Autodesk Fusion 360 part; units mm, degrees
note: some values were not read from the file. Set by a fixed rule: which sketch regions a step uses.
(part 4 of 10)
  spline S19 degree 5 poles (-4.5069, -15.3521) (-4.5055, -15.3505) (-4.5027, -15.3473) (-4.4985, -15.3425) (-4.493, -15.3361) (-4.486, -15.3281) (-4.4791, -15.3201) (-4.4722, -15.3121) (-4.4654, -15.3042) (-4.4586, -15.2962) (-4.4518, -15.2883) (-4.445, -15.2803) (-4.4383, -15.2724) (-4.4316, -15.2645) (-4.4249, -15.2565) (-4.4183, -15.2486) (-4.4117, -15.2407) (-4.4051, -15.2329) (-4.3985, -15.225) (-4.392, -15.2171) (-4.3855, -15.2093) (-4.3791, -15.2014) (-4.3726, -15.1936) (-4.3662, -15.1858) (-4.3599, -15.178) (-4.3535, -15.1702) (-4.3472, -15.1624) (-4.3409, -15.1546) (-4.3347, -15.1468) (-4.3285, -15.1391) (-4.3223, -15.1313) (-4.3161, -15.1236) (-4.31, -15.1159) (-4.3039, -15.1082) (-4.2978, -15.1005) (-4.2918, -15.0928) (-4.2858, -15.0851) (-4.2798, -15.0775) (-4.2738, -15.0698) (-4.2679, -15.0622) (-4.262, -15.0546) (-4.2562, -15.047) (-4.2503, -15.0394) (-4.2445, -15.0318) (-4.2388, -15.0242) (-4.233, -15.0167) (-4.2273, -15.0092) (-4.2216, -15.0016) (-4.216, -14.9941) (-4.2104, -14.9866) (-4.2048, -14.9791) (-4.1992, -14.9717) (-4.1937, -14.9642) (-4.1882, -14.9568) (-4.1827, -14.9494) (-4.1773, -14.942) (-4.1719, -14.9346) (-4.1665, -14.9272) (-4.1612, -14.9198) (-4.1559, -14.9125) (-4.1506, -14.9052) (-4.1453, -14.8978) (-4.1401, -14.8905) (-4.1349, -14.8833) (-4.1297, -14.876) (-4.1246, -14.8687) (-4.1195, -14.8615) (-4.1144, -14.8543) (-4.1094, -14.8471) (-4.1044, -14.8399) (-4.0994, -14.8328) (-4.0944, -14.8256) (-4.0895, -14.8185) (-4.0846, -14.8114) (-4.0798, -14.8043) (-4.0749, -14.7972) (-4.0701, -14.7901) (-4.0654, -14.7831) (-4.0606, -14.7761) (-4.0559, -14.7691) (-4.0512, -14.7621) (-4.0466, -14.7551) (-4.042, -14.7482) (-4.0374, -14.7413) (-4.0328, -14.7344) (-4.0283, -14.7275) (-4.0238, -14.7206) (-4.0193, -14.7138) (-4.0149, -14.707) (-4.0105, -14.7002) (-4.0061, -14.6934) (-4.0018, -14.6866) (-3.9974, -14.6799) (-3.9932, -14.6731) (-3.9889, -14.6665) (-3.9847, -14.6598) (-3.9805, -14.6531) (-3.9763, -14.6465) (-3.9722, -14.6399) (-3.9681, -14.6333) (-3.964, -14.6267) (-3.96, -14.6202) (-3.9559, -14.6137) (-3.952, -14.6072) (-3.948, -14.6007) (-3.9441, -14.5942) (-3.9402, -14.5878) (-3.9363, -14.5814) (-3.9325, -14.575) (-3.9287, -14.5687) (-3.9249, -14.5623) (-3.9212, -14.556) (-3.9175, -14.5497) (-3.9138, -14.5435) (-3.9101, -14.5373) (-3.9065, -14.5311) (-3.9029, -14.5249) (-3.8993, -14.5187) (-3.8958, -14.5126) (-3.8923, -14.5065) (-3.8888, -14.5004) (-3.8854, -14.4944) (-3.882, -14.4883) (-3.8786, -14.4824) (-3.8752, -14.4764) (-3.8719, -14.4704) (-3.8686, -14.4645) (-3.8654, -14.4587) (-3.8621, -14.4528) (-3.8589, -14.447) (-3.8558, -14.4412) (-3.8526, -14.4354) (-3.8495, -14.4297) (-3.8464, -14.424) (-3.8434, -14.4183) (-3.8403, -14.4126) (-3.8373, -14.407) (-3.8344, -14.4014) (-3.8314, -14.3959) (-3.8285, -14.3903) (-3.8257, -14.3848) (-3.8228, -14.3794) (-3.82, -14.3739) (-3.8172, -14.3685) (-3.8144, -14.3632) (-3.8117, -14.3578) (-3.809, -14.3525) (-3.8063, -14.3473) (-3.8037, -14.342) (-3.8011, -14.3368) (-3.7985, -14.3316) (-3.796, -14.3265) (-3.7934, -14.3214) (-3.791, -14.3163) (-3.7885, -14.3113) (-3.7861, -14.3063) (-3.7836, -14.3013) (-3.7813, -14.2964) (-3.7789, -14.2915) (-3.7766, -14.2867) (-3.7743, -14.2819) (-3.7721, -14.2771) (-3.7698, -14.2723) (-3.7676, -14.2676) (-3.7655, -14.263) (-3.7633, -14.2583) (-3.7612, -14.2537) (-3.7591, -14.2492) (-3.7571, -14.2447) (-3.755, -14.2402) (-3.753, -14.2358) (-3.7511, -14.2314) (-3.7491, -14.227) (-3.7472, -14.2227) (-3.7453, -14.2185) (-3.7435, -14.2142) (-3.7416, -14.21) (-3.7398, -14.2059) (-3.7381, -14.2018) (-3.7363, -14.1977) (-3.7346, -14.1937) (-3.7329, -14.1898) (-3.7313, -14.1858) (-3.7296, -14.1819) (-3.728, -14.1781) (-3.7265, -14.1743) (-3.7249, -14.1706) (-3.7234, -14.1669) (-3.7219, -14.1632) (-3.7204, -14.1596) (-3.719, -14.1561) (-3.7176, -14.1525) (-3.7162, -14.1491) (-3.7149, -14.1457) (-3.7136, -14.1423) (-3.7123, -14.139) (-3.711, -14.1357) (-3.7097, -14.1325) (-3.7085, -14.1293) (-3.7073, -14.1262) (-3.7062, -14.1232) (-3.7051, -14.1202) (-3.704, -14.1172) (-3.7029, -14.1143) (-3.7018, -14.1114) (-3.7008, -14.1086) (-3.6998, -14.1059) (-3.6988, -14.1032) (-3.6979, -14.1006) (-3.697, -14.098) (-3.6961, -14.0955) (-3.6952, -14.093) (-3.6944, -14.0906) (-3.6936, -14.0883) (-3.6928, -14.086) (-3.692, -14.0838) (-3.6913, -14.0816) (-3.6906, -14.0795) (-3.6899, -14.0775) (-3.6892, -14.0755) (-3.6886, -14.0736) (-3.688, -14.0717) (-3.6874, -14.0699) (-3.6869, -14.0682) (-3.6863, -14.0665) (-3.6858, -14.0649) (-3.6853, -14.0634) (-3.6849, -14.0619) (-3.6845, -14.0606) (-3.6841, -14.0592) (-3.6837, -14.058) (-3.6833, -14.0568) (-3.683, -14.0557) (-3.6827, -14.0546) (-3.6824, -14.0537) (-3.6821, -14.0528) (-3.6819, -14.0519) (-3.6817, -14.0512) (-3.6815, -14.0505) (-3.6813, -14.0499) (-3.6812, -14.0494) (-3.6811, -14.0491) (-3.681, -14.0488) (-3.681, -14.0487) (-3.681, -14.0486) knots -1 -1 -1 -1 -1 -1 -0.99583333 -0.99166667 -0.9875 -0.98333333 -0.97916667 -0.975 -0.97083333 -0.96666667 -0.9625 -0.95833333 -0.95416667 -0.95 -0.94583333 -0.94166667 -0.9375 -0.93333333 -0.92916667 -0.925 -0.92083333 -0.91666667 -0.9125 -0.90833333 -0.90416667 -0.9 -0.89583333 -0.89166667 -0.8875 -0.88333333 -0.87916667 -0.875 -0.87083333 -0.86666667 -0.8625 -0.85833333 -0.85416667 -0.85 -0.84583333 -0.84166667 -0.8375 -0.83333333 -0.82916667 -0.825 -0.82083333 -0.81666667 -0.8125 -0.80833333 -0.80416667 -0.8 -0.79583333 -0.79166667 -0.7875 -0.78333333 -0.77916667 -0.775 -0.77083333 -0.76666667 -0.7625 -0.75833333 -0.75416667 -0.75 -0.74583333 -0.74166667 -0.7375 -0.73333333 -0.72916667 -0.725 -0.72083333 -0.71666667 -0.7125 -0.70833333 -0.70416667 -0.7 -0.69583333 -0.69166667 -0.6875 -0.68333333 -0.67916667 -0.675 -0.67083333 -0.66666667 -0.6625 -0.65833333 -0.65416667 -0.65 -0.64583333 -0.64166667 -0.6375 -0.63333333 -0.62916667 -0.625 -0.62083333 -0.61666667 -0.6125 -0.60833333 -0.60416667 -0.6 -0.59583333 -0.59166667 -0.5875 -0.58333333 -0.57916667 -0.575 -0.57083333 -0.56666667 -0.5625 -0.55833333 -0.55416667 -0.55 -0.54583333 -0.54166667 -0.5375 -0.53333333 -0.52916667 -0.525 -0.52083333 -0.51666667 -0.5125 -0.50833333 -0.50416667 -0.5 -0.49583333 -0.49166667 -0.4875 -0.48333333 -0.47916667 -0.475 -0.47083333 -0.46666667 -0.4625 -0.45833333 -0.45416667 -0.45 -0.44583333 -0.44166667 -0.4375 -0.43333333 -0.42916667 -0.425 -0.42083333 -0.41666667 -0.4125 -0.40833333 -0.40416667 -0.4 -0.39583333 -0.39166667 -0.3875 -0.38333333 -0.37916667 -0.375 -0.37083333 -0.36666667 -0.3625 -0.35833333 -0.35416667 -0.35 -0.34583333 -0.34166667 -0.3375 -0.33333333 -0.32916667 -0.325 -0.32083333 -0.31666667 -0.3125 -0.30833333 -0.30416667 -0.3 -0.29583333 -0.29166667 -0.2875 -0.28333333 -0.27916667 -0.275 -0.27083333 -0.26666667 -0.2625 -0.25833333 -0.25416667 -0.25 -0.24583333 -0.24166667 -0.2375 -0.23333333 -0.22916667 -0.225 -0.22083333 -0.21666667 -0.2125 -0.20833333 -0.20416667 -0.2 -0.19583333 -0.19166667 -0.1875 -0.18333333 -0.17916667 -0.175 -0.17083333 -0.16666667 -0.1625 -0.15833333 -0.15416667 -0.15 -0.14583333 -0.14166667 -0.1375 -0.13333333 -0.12916667 -0.125 -0.12083333 -0.11666667 -0.1125 -0.10833333 -0.10416667 -0.1 -0.09583333 -0.09166667 -0.0875 -0.08333333 -0.07916667 -0.075 -0.07083333 -0.06666667 -0.0625 -0.05833333 -0.05416667 -0.05 -0.04583333 -0.04166667 -0.0375 -0.03333333 -0.02916667 -0.025 -0.02083333 -0.01666667 -0.0125 -0.00833333 -0.00416667 0 0 0 0 0 0
  arc A26 (8.5938, 10.7336) -> (7.5526, 11.49) centre (0, 0) ccw
  arc A27 (8.3931, 13.6219) -> (7.6003, 14.0796) centre (0, 0) ccw
  line L59 (2.3513, -14.3306) -> (2.2262, -13.5686)
  line L60 (9.0768, 11.3369) -> (9.0764, 11.3364)
  line L61 (11.235, 9.2016) -> (10.6376, 8.7123)
  line L62 (3.6808, -14.048) -> (3.681, -14.0486)
  arc A28 (10.6376, 8.7123) -> (9.7765, 9.6687) centre (0, 0) ccw
  line L63 (7.5526, 11.49) -> (7.9768, 12.1353)
  arc A29 (13.208, 9.0304) -> (12.6699, 9.771) centre (0, 0) ccw
  line L64 (0.6435, -13.7349) -> (0.6796, -14.5063)
  line L65 (10.3255, 10.2117) -> (10.326, 10.2121)
  spline S20 degree 5 poles (10.3616, 12.1917) (10.3596, 12.1908) (10.3558, 12.189) (10.35, 12.1863) (10.3423, 12.1828) (10.3327, 12.1783) (10.3231, 12.1738) (10.3136, 12.1693) (10.3041, 12.1648) (10.2946, 12.1603) (10.2852, 12.1558) (10.2758, 12.1513) (10.2664, 12.1468) (10.2571, 12.1423) (10.2478, 12.1378) (10.2385, 12.1332) (10.2292, 12.1287) (10.22, 12.1242) (10.2108, 12.1197) (10.2017, 12.1151) (10.1925, 12.1106) (10.1834, 12.1061) (10.1744, 12.1015) (10.1654, 12.097) (10.1564, 12.0924) (10.1474, 12.0879) (10.1385, 12.0834) (10.1296, 12.0788) (10.1207, 12.0743) (10.1119, 12.0697) (10.1031, 12.0651) (10.0943, 12.0606) (10.0855, 12.056) (10.0768, 12.0515) (10.0682, 12.0469) (10.0595, 12.0423) (10.0509, 12.0378) (10.0423, 12.0332) (10.0338, 12.0287) (10.0253, 12.0241) (10.0168, 12.0195) (10.0084, 12.015) (9.9999, 12.0104) (9.9916, 12.0058) (9.9832, 12.0013) (9.9749, 11.9967) (9.9666, 11.9921) (9.9584, 11.9876) (9.9502, 11.983) (9.942, 11.9785) (9.9338, 11.9739) (9.9257, 11.9693) (9.9176, 11.9648) (9.9096, 11.9602) (9.9016, 11.9557) (9.8936, 11.9511) (9.8857, 11.9465) (9.8777, 11.942) (9.8699, 11.9374) (9.862, 11.9329) (9.8542, 11.9283) (9.8464, 11.9238) (9.8387, 11.9193) (9.831, 11.9147) (9.8233, 11.9102) (9.8157, 11.9056) (9.8081, 11.9011) (9.8005, 11.8966) (9.793, 11.8921) (9.7855, 11.8875) (9.778, 11.883) (9.7706, 11.8785) (9.7632, 11.874) (9.7558, 11.8695) (9.7485, 11.865) (9.7412, 11.8605) (9.7339, 11.856) (9.7267, 11.8515) (9.7195, 11.847) (9.7124, 11.8425) (9.7053, 11.8381) (9.6982, 11.8336) (9.6912, 11.8291) (9.6841, 11.8247) (9.6772, 11.8202) (9.6702, 11.8158) (9.6633, 11.8113) (9.6565, 11.8069) (9.6496, 11.8025) (9.6428, 11.798) (9.6361, 11.7936) (9.6294, 11.7892) (9.6227, 11.7848) (9.616, 11.7804) (9.6094, 11.776) (9.6028, 11.7717) (9.5963, 11.7673) (9.5898, 11.7629) (9.5833, 11.7586) (9.5769, 11.7542) (9.5705, 11.7499) (9.5642, 11.7455) (9.5578, 11.7412) (9.5516, 11.7369) (9.5453, 11.7326) (9.5391, 11.7283) (9.5329, 11.724) (9.5268, 11.7197) (9.5207, 11.7155) (9.5146, 11.7112) (9.5086, 11.707) (9.5026, 11.7027) (9.4967, 11.6985) (9.4908, 11.6943) (9.4849, 11.6901) (9.4791, 11.6859) (9.4733, 11.6817) (9.4675, 11.6775) (9.4618, 11.6733) (9.4561, 11.6692) (9.4505, 11.6651) (9.4449, 11.6609) (9.4393, 11.6568) (9.4338, 11.6527) (9.4283, 11.6486) (9.4228, 11.6446) (9.4174, 11.6405) (9.412, 11.6365) (9.4067, 11.6324) (9.4014, 11.6284) (9.3962, 11.6244) (9.3909, 11.6204) (9.3858, 11.6164) (9.3806, 11.6125) (9.3755, 11.6085) (9.3705, 11.6046) (9.3654, 11.6007) (9.3605, 11.5968) (9.3555, 11.5929) (9.3506, 11.589) (9.3457, 11.5852) (9.3409, 11.5813) (9.3361, 11.5775) (9.3314, 11.5737) (9.3267, 11.5699) (9.322, 11.5662) (9.3174, 11.5624) (9.3128, 11.5587) (9.3083, 11.555) (9.3038, 11.5513) (9.2993, 11.5476) (9.2949, 11.544) (9.2905, 11.5403) (9.2862, 11.5367) (9.2819, 11.5331) (9.2776, 11.5295) (9.2734, 11.526) (9.2692, 11.5224) (9.2651, 11.5189) (9.261, 11.5154) (9.257, 11.512) (9.253, 11.5085) (9.249, 11.5051) (9.2451, 11.5017) (9.2412, 11.4983) (9.2373, 11.495) (9.2335, 11.4916) (9.2298, 11.4883) (9.2261, 11.485) (9.2224, 11.4818) (9.2188, 11.4785) (9.2152, 11.4753) (9.2116, 11.4721) (9.2081, 11.469) (9.2047, 11.4658) (9.2013, 11.4627) (9.1979, 11.4597) (9.1946, 11.4566) (9.1913, 11.4536) (9.188, 11.4506) (9.1848, 11.4476) (9.1817, 11.4447) (9.1786, 11.4418) (9.1755, 11.4389) (9.1725, 11.436) (9.1695, 11.4332) (9.1666, 11.4304) (9.1637, 11.4276) (9.1608, 11.4249) (9.158, 11.4222) (9.1553, 11.4195) (9.1526, 11.4169) (9.1499, 11.4143) (9.1473, 11.4117) (9.1447, 11.4092) (9.1422, 11.4067) (9.1397, 11.4042) (9.1372, 11.4018) (9.1348, 11.3994) (9.1325, 11.397) (9.1302, 11.3947) (9.1279, 11.3924) (9.1257, 11.3902) (9.1235, 11.388) (9.1214, 11.3858) (9.1194, 11.3836) (9.1173, 11.3815) (9.1153, 11.3795) (9.1134, 11.3775) (9.1115, 11.3755) (9.1097, 11.3735) (9.1079, 11.3717) (9.1062, 11.3698) (9.1045, 11.368) (9.1028, 11.3662) (9.1012, 11.3645) (9.0997, 11.3628) (9.0982, 11.3612) (9.0967, 11.3596) (9.0953, 11.3581) (9.0939, 11.3566) (9.0926, 11.3551) (9.0914, 11.3537) (9.0902, 11.3524) (9.089, 11.3511) (9.0879, 11.3498) (9.0868, 11.3486) (9.0858, 11.3475) (9.0849, 11.3464) (9.084, 11.3453) (9.0831, 11.3443) (9.0823, 11.3434) (9.0815, 11.3425) (9.0808, 11.3417) (9.0802, 11.3409) (9.0796, 11.3402) (9.079, 11.3395) (9.0785, 11.3389) (9.0781, 11.3384) (9.0777, 11.3379) (9.0773, 11.3375) (9.0771, 11.3372) (9.0769, 11.337) (9.0769, 11.3369) (9.0768, 11.3369) knots -1 -1 -1 -1 -1 -1 -0.99583333 -0.99166667 -0.9875 -0.98333333 -0.97916667 -0.975 -0.97083333 -0.96666667 -0.9625 -0.95833333 -0.95416667 -0.95 -0.94583333 -0.94166667 -0.9375 -0.93333333 -0.92916667 -0.925 -0.92083333 -0.91666667 -0.9125 -0.90833333 -0.90416667 -0.9 -0.89583333 -0.89166667 -0.8875 -0.88333333 -0.87916667 -0.875 -0.87083333 -0.86666667 -0.8625 -0.85833333 -0.85416667 -0.85 -0.84583333 -0.84166667 -0.8375 -0.83333333 -0.82916667 -0.825 -0.82083333 -0.81666667 -0.8125 -0.80833333 -0.80416667 -0.8 -0.79583333 -0.79166667 -0.7875 -0.78333333 -0.77916667 -0.775 -0.77083333 -0.76666667 -0.7625 -0.75833333 -0.75416667 -0.75 -0.74583333 -0.74166667 -0.7375 -0.73333333 -0.72916667 -0.725 -0.72083333 -0.71666667 -0.7125 -0.70833333 -0.70416667 -0.7 -0.69583333 -0.69166667 -0.6875 -0.68333333 -0.67916667 -0.675 -0.67083333 -0.66666667 -0.6625 -0.65833333 -0.65416667 -0.65 -0.64583333 -0.64166667 -0.6375 -0.63333333 -0.62916667 -0.625 -0.62083333 -0.61666667 -0.6125 -0.60833333 -0.60416667 -0.6 -0.59583333 -0.59166667 -0.5875 -0.58333333 -0.57916667 -0.575 -0.57083333 -0.56666667 -0.5625 -0.55833333 -0.55416667 -0.55 -0.54583333 -0.54166667 -0.5375 -0.53333333 -0.52916667 -0.525 -0.52083333 -0.51666667 -0.5125 -0.50833333 -0.50416667 -0.5 -0.49583333 -0.49166667 -0.4875 -0.48333333 -0.47916667 -0.475 -0.47083333 -0.46666667 -0.4625 -0.45833333 -0.45416667 -0.45 -0.44583333 -0.44166667 -0.4375 -0.43333333 -0.42916667 -0.425 -0.42083333 -0.41666667 -0.4125 -0.40833333 -0.40416667 -0.4 -0.39583333 -0.39166667 -0.3875 -0.38333333 -0.37916667 -0.375 -0.37083333 -0.36666667 -0.3625 -0.35833333 -0.35416667 -0.35 -0.34583333 -0.34166667 -0.3375 -0.33333333 -0.32916667 -0.325 -0.32083333 -0.31666667 -0.3125 -0.30833333 -0.30416667 -0.3 -0.29583333 -0.29166667 -0.2875 -0.28333333 -0.27916667 -0.275 -0.27083333 -0.26666667 -0.2625 -0.25833333 -0.25416667 -0.25 -0.24583333 -0.24166667 -0.2375 -0.23333333 -0.22916667 -0.225 -0.22083333 -0.21666667 -0.2125 -0.20833333 -0.20416667 -0.2 -0.19583333 -0.19166667 -0.1875 -0.18333333 -0.17916667 -0.175 -0.17083333 -0.16666667 -0.1625 -0.15833333 -0.15416667 -0.15 -0.14583333 -0.14166667 -0.1375 -0.13333333 -0.12916667 -0.125 -0.12083333 -0.11666667 -0.1125 -0.10833333 -0.10416667 -0.1 -0.09583333 -0.09166667 -0.0875 -0.08333333 -0.07916667 -0.075 -0.07083333 -0.06666667 -0.0625 -0.05833333 -0.05416667 -0.05 -0.04583333 -0.04166667 -0.0375 -0.03333333 -0.02916667 -0.025 -0.02083333 -0.01666667 -0.0125 -0.00833333 -0.00416667 0 0 0 0 0 0
  line L66 (6.5211, -12.9757) -> (6.5214, -12.9763)
  spline S21 degree 5 poles (-15.9935, -0.4577) (-15.9915, -0.4585) (-15.9876, -0.4602) (-15.9817, -0.4627) (-15.9739, -0.466) (-15.9641, -0.4702) (-15.9544, -0.4743) (-15.9447, -0.4784) (-15.935, -0.4824) (-15.9253, -0.4864) (-15.9157, -0.4904) (-15.906, -0.4944) (-15.8964, -0.4984) (-15.8868, -0.5023) (-15.8772, -0.5062) (-15.8676, -0.5101) (-15.8581, -0.5139) (-15.8486, -0.5177) (-15.839, -0.5215) (-15.8295, -0.5253) (-15.8201, -0.529) (-15.8106, -0.5328) (-15.8012, -0.5365) (-15.7918, -0.5401) (-15.7824, -0.5438) (-15.773, -0.5474) (-15.7636, -0.551) (-15.7543, -0.5546) (-15.745, -0.5581) (-15.7357, -0.5616) (-15.7264, -0.5651) (-15.7172, -0.5686) (-15.7079, -0.572) (-15.6987, -0.5755) (-15.6895, -0.5789) (-15.6803, -0.5822) (-15.6712, -0.5856) (-15.6621, -0.5889) (-15.653, -0.5922) (-15.6439, -0.5955) (-15.6348, -0.5987) (-15.6258, -0.6019) (-15.6167, -0.6051) (-15.6077, -0.6083) (-15.5988, -0.6114) (-15.5898, -0.6146) (-15.5809, -0.6177) (-15.572, -0.6207) (-15.5631, -0.6238) (-15.5542, -0.6268) (-15.5454, -0.6298) (-15.5365, -0.6328) (-15.5278, -0.6358) (-15.519, -0.6387) (-15.5102, -0.6416) (-15.5015, -0.6445) (-15.4928, -0.6473) (-15.4841, -0.6502) (-15.4755, -0.653) (-15.4668, -0.6558) (-15.4582, -0.6585) (-15.4497, -0.6613) (-15.4411, -0.664) (-15.4326, -0.6667) (-15.4241, -0.6693) (-15.4156, -0.672) (-15.4071, -0.6746) (-15.3987, -0.6772) (-15.3903, -0.6797) (-15.3819, -0.6823) (-15.3736, -0.6848) (-15.3652, -0.6873) (-15.3569, -0.6898) (-15.3487, -0.6923) (-15.3404, -0.6947) (-15.3322, -0.6971) (-15.324, -0.6995) (-15.3158, -0.7018) (-15.3077, -0.7042) (-15.2996, -0.7065) (-15.2915, -0.7088) (-15.2834, -0.7111) (-15.2754, -0.7133) (-15.2674, -0.7155) (-15.2594, -0.7177) (-15.2515, -0.7199) (-15.2436, -0.7221) (-15.2357, -0.7242) (-15.2278, -0.7263) (-15.22, -0.7284) (-15.2122, -0.7305) (-15.2044, -0.7325) (-15.1967, -0.7345) (-15.1889, -0.7365) (-15.1813, -0.7385) (-15.1736, -0.7405) (-15.166, -0.7424) (-15.1584, -0.7443) (-15.1508, -0.7462) (-15.1433, -0.7481) (-15.1358, -0.7499) (-15.1283, -0.7517) (-15.1209, -0.7535) (-15.1135, -0.7553) (-15.1061, -0.7571) (-15.0987, -0.7588) (-15.0914, -0.7605) (-15.0841, -0.7622) (-15.0769, -0.7639) (-15.0697, -0.7656) (-15.0625, -0.7672) (-15.0553, -0.7688) (-15.0482, -0.7704) (-15.0411, -0.772) (-15.0341, -0.7735) (-15.027, -0.775) (-15.02, -0.7766) (-15.0131, -0.778) (-15.0062, -0.7795) (-14.9993, -0.781) (-14.9924, -0.7824) (-14.9856, -0.7838) (-14.9788, -0.7852) (-14.9721, -0.7865) (-14.9654, -0.7879) (-14.9587, -0.7892) (-14.9521, -0.7905) (-14.9455, -0.7918) (-14.9389, -0.7931) (-14.9324, -0.7943) (-14.9259, -0.7955) (-14.9194, -0.7967) (-14.913, -0.7979) (-14.9066, -0.7991) (-14.9003, -0.8002) (-14.8939, -0.8014) (-14.8877, -0.8025) (-14.8814, -0.8036) (-14.8753, -0.8047) (-14.8691, -0.8057) (-14.863, -0.8067) (-14.8569, -0.8078) (-14.8509, -0.8088) (-14.8449, -0.8097) (-14.8389, -0.8107) (-14.833, -0.8117) (-14.8271, -0.8126) (-14.8213, -0.8135) (-14.8155, -0.8144) (-14.8097, -0.8153) (-14.804, -0.8161) (-14.7983, -0.817) (-14.7927, -0.8178) (-14.7871, -0.8186) (-14.7816, -0.8194) (-14.7761, -0.8201) (-14.7706, -0.8209) (-14.7652, -0.8216) (-14.7598, -0.8224) (-14.7545, -0.8231) (-14.7492, -0.8237) (-14.7439, -0.8244) (-14.7387, -0.8251) (-14.7336, -0.8257) (-14.7285, -0.8263) (-14.7234, -0.8269) (-14.7184, -0.8275) (-14.7134, -0.8281) (-14.7085, -0.8287) (-14.7036, -0.8292) (-14.6988, -0.8298) (-14.694, -0.8303) (-14.6893, -0.8308) (-14.6846, -0.8313) (-14.6799, -0.8317) (-14.6753, -0.8322) (-14.6708, -0.8326) (-14.6663, -0.8331) (-14.6618, -0.8335) (-14.6574, -0.8339) (-14.6531, -0.8343) (-14.6488, -0.8347) (-14.6446, -0.835) (-14.6404, -0.8354) (-14.6362, -0.8357) (-14.6321, -0.836) (-14.6281, -0.8363) (-14.6241, -0.8366) (-14.6202, -0.8369) (-14.6163, -0.8372) (-14.6124, -0.8375) (-14.6087, -0.8377) (-14.605, -0.838) (-14.6013, -0.8382) (-14.5977, -0.8384) (-14.5941, -0.8386) (-14.5906, -0.8388) (-14.5872, -0.839) (-14.5838, -0.8392) (-14.5805, -0.8393) (-14.5772, -0.8395) (-14.574, -0.8396) (-14.5708, -0.8398) (-14.5677, -0.8399) (-14.5647, -0.84) (-14.5617, -0.8401) (-14.5588, -0.8402) (-14.556, -0.8403) (-14.5532, -0.8404) (-14.5504, -0.8405) (-14.5478, -0.8406) (-14.5452, -0.8406) (-14.5426, -0.8407) (-14.5401, -0.8407) (-14.5377, -0.8408) (-14.5354, -0.8408) (-14.5331, -0.8408) (-14.5309, -0.8409) (-14.5287, -0.8409) (-14.5266, -0.8409) (-14.5246, -0.8409) (-14.5226, -0.8409) (-14.5208, -0.8409) (-14.519, -0.8409) (-14.5172, -0.8409) (-14.5155, -0.8409) (-14.5139, -0.8409) (-14.5124, -0.8408) (-14.5109, -0.8408) (-14.5096, -0.8408) (-14.5082, -0.8408) (-14.507, -0.8407) (-14.5058, -0.8407) (-14.5048, -0.8407) (-14.5037, -0.8407) (-14.5028, -0.8406) (-14.502, -0.8406) (-14.5012, -0.8406) (-14.5005, -0.8406) (-14.4999, -0.8405) (-14.4993, -0.8405) (-14.499, -0.8405) (-14.4987, -0.8405) (-14.4986, -0.8405) (-14.4985, -0.8405) knots -1 -1 -1 -1 -1 -1 -0.99583333 -0.99166667 -0.9875 -0.98333333 -0.97916667 -0.975 -0.97083333 -0.96666667 -0.9625 -0.95833333 -0.95416667 -0.95 -0.94583333 -0.94166667 -0.9375 -0.93333333 -0.92916667 -0.925 -0.92083333 -0.91666667 -0.9125 -0.90833333 -0.90416667 -0.9 -0.89583333 -0.89166667 -0.8875 -0.88333333 -0.87916667 -0.875 -0.87083333 -0.86666667 -0.8625 -0.85833333 -0.85416667 -0.85 -0.84583333 -0.84166667 -0.8375 -0.83333333 -0.82916667 -0.825 -0.82083333 -0.81666667 -0.8125 -0.80833333 -0.80416667 -0.8 -0.79583333 -0.79166667 -0.7875 -0.78333333 -0.77916667 -0.775 -0.77083333 -0.76666667 -0.7625 -0.75833333 -0.75416667 -0.75 -0.74583333 -0.74166667 -0.7375 -0.73333333 -0.72916667 -0.725 -0.72083333 -0.71666667 -0.7125 -0.70833333 -0.70416667 -0.7 -0.69583333 -0.69166667 -0.6875 -0.68333333 -0.67916667 -0.675 -0.67083333 -0.66666667 -0.6625 -0.65833333 -0.65416667 -0.65 -0.64583333 -0.64166667 -0.6375 -0.63333333 -0.62916667 -0.625 -0.62083333 -0.61666667 -0.6125 -0.60833333 -0.60416667 -0.6 -0.59583333 -0.59166667 -0.5875 -0.58333333 -0.57916667 -0.575 -0.57083333 -0.56666667 -0.5625 -0.55833333 -0.55416667 -0.55 -0.54583333 -0.54166667 -0.5375 -0.53333333 -0.52916667 -0.525 -0.52083333 -0.51666667 -0.5125 -0.50833333 -0.50416667 -0.5 -0.49583333 -0.49166667 -0.4875 -0.48333333 -0.47916667 -0.475 -0.47083333 -0.46666667 -0.4625 -0.45833333 -0.45416667 -0.45 -0.44583333 -0.44166667 -0.4375 -0.43333333 -0.42916667 -0.425 -0.42083333 -0.41666667 -0.4125 -0.40833333 -0.40416667 -0.4 -0.39583333 -0.39166667 -0.3875 -0.38333333 -0.37916667 -0.375 -0.37083333 -0.36666667 -0.3625 -0.35833333 -0.35416667 -0.35 -0.34583333 -0.34166667 -0.3375 -0.33333333 -0.32916667 -0.325 -0.32083333 -0.31666667 -0.3125 -0.30833333 -0.30416667 -0.3 -0.29583333 -0.29166667 -0.2875 -0.28333333 -0.27916667 -0.275 -0.27083333 -0.26666667 -0.2625 -0.25833333 -0.25416667 -0.25 -0.24583333 -0.24166667 -0.2375 -0.23333333 -0.22916667 -0.225 -0.22083333 -0.21666667 -0.2125 -0.20833333 -0.20416667 -0.2 -0.19583333 -0.19166667 -0.1875 -0.18333333 -0.17916667 -0.175 -0.17083333 -0.16666667 -0.1625 -0.15833333 -0.15416667 -0.15 -0.14583333 -0.14166667 -0.1375 -0.13333333 -0.12916667 -0.125 -0.12083333 -0.11666667 -0.1125 -0.10833333 -0.10416667 -0.1 -0.09583333 -0.09166667 -0.0875 -0.08333333 -0.07916667 -0.075 -0.07083333 -0.06666667 -0.0625 -0.05833333 -0.05416667 -0.05 -0.04583333 -0.04166667 -0.0375 -0.03333333 -0.02916667 -0.025 -0.02083333 -0.01666667 -0.0125 -0.00833333 -0.00416667 0 0 0 0 0 0
  line L67 (-14.4979, -0.8404) -> (-13.727, -0.7957)
  arc A30 (4.9987, -12.8092) -> (6.1743, -12.2858) centre (0, 0) ccw
  spline S22 degree 5 poles (5.3776, -15.0692) (5.3777, -15.0671) (5.3781, -15.0629) (5.3787, -15.0565) (5.3794, -15.0481) (5.3804, -15.0375) (5.3813, -15.027) (5.3821, -15.0165) (5.383, -15.006) (5.3838, -14.9956) (5.3846, -14.9851) (5.3854, -14.9747) (5.3862, -14.9644) (5.387, -14.954) (5.3877, -14.9437) (5.3885, -14.9334) (5.3892, -14.9231) (5.3899, -14.9129) (5.3905, -14.9027) (5.3912, -14.8925) (5.3918, -14.8823) (5.3924, -14.8722) (5.393, -14.862) (5.3936, -14.852) (5.3942, -14.8419) (5.3947, -14.8319) (5.3953, -14.8218) (5.3958, -14.8119) (5.3963, -14.8019) (5.3967, -14.792) (5.3972, -14.7821) (5.3976, -14.7722) (5.3981, -14.7624) (5.3985, -14.7525) (5.3988, -14.7427) (5.3992, -14.733) (5.3996, -14.7232) (5.3999, -14.7135) (5.4002, -14.7038) (5.4005, -14.6942) (5.4008, -14.6846) (5.4011, -14.675) (5.4013, -14.6654) (5.4016, -14.6559) (5.4018, -14.6464) (5.402, -14.6369) (5.4022, -14.6274) (5.4024, -14.618) (5.4025, -14.6086) (5.4027, -14.5992) (5.4028, -14.5899) (5.4029, -14.5806) (5.403, -14.5713) (5.4031, -14.5621) (5.4031, -14.5528) (5.4032, -14.5437) (5.4032, -14.5345) (5.4032, -14.5254) (5.4032, -14.5163) (5.4032, -14.5072) (5.4031, -14.4982) (5.4031, -14.4892) (5.403, -14.4802) (5.403, -14.4712) (5.4029, -14.4623) (5.4028, -14.4535) (5.4026, -14.4446) (5.4025, -14.4358) (5.4023, -14.427) (5.4022, -14.4182) (5.402, -14.4095) (5.4018, -14.4008) (5.4016, -14.3922) (5.4014, -14.3835) (5.4011, -14.3749) (5.4009, -14.3664) (5.4006, -14.3578) (5.4003, -14.3493) (5.4001, -14.3409) (5.3998, -14.3325) (5.3994, -14.3241) (5.3991, -14.3157) (5.3988, -14.3074) (5.3984, -14.2991) (5.398, -14.2908) (5.3976, -14.2826) (5.3973, -14.2744) (5.3968, -14.2662) (5.3964, -14.2581) (5.396, -14.25) (5.3955, -14.2419) (5.3951, -14.2339) (5.3946, -14.2259) (5.3941, -14.2179) (5.3936, -14.21) (5.3931, -14.2021) (5.3926, -14.1943) (5.3921, -14.1865) (5.3915, -14.1787) (5.391, -14.171) (5.3904, -14.1632) (5.3899, -14.1556) (5.3893, -14.1479) (5.3887, -14.1403) (5.3881, -14.1328) (5.3874, -14.1253) (5.3868, -14.1178) (5.3862, -14.1103) (5.3855, -14.1029) (5.3849, -14.0955) (5.3842, -14.0882) (5.3835, -14.0809) (5.3828, -14.0736) (5.3821, -14.0664) (5.3814, -14.0592) (5.3807, -14.0521) (5.38, -14.0449) (5.3793, -14.0379) (5.3785, -14.0308) (5.3778, -14.0238) (5.377, -14.0169) (5.3762, -14.01) (5.3755, -14.0031) (5.3747, -13.9963) (5.3739, -13.9895) (5.3731, -13.9827) (5.3723, -13.976) (5.3714, -13.9693) (5.3706, -13.9627) (5.3698, -13.9561) (5.3689, -13.9495) (5.3681, -13.943) (5.3672, -13.9365) (5.3664, -13.9301) (5.3655, -13.9237) (5.3646, -13.9173) (5.3638, -13.911) (5.3629, -13.9048) (5.362, -13.8986) (5.3611, -13.8924) (5.3602, -13.8862) (5.3593, -13.8801) (5.3583, -13.8741) (5.3574, -13.8681) (5.3565, -13.8621) (5.3556, -13.8562) (5.3546, -13.8503) (5.3537, -13.8445) (5.3528, -13.8387) (5.3518, -13.833) (5.3509, -13.8273) (5.3499, -13.8216) (5.3489, -13.816) (5.348, -13.8104) (5.347, -13.8049) (5.3461, -13.7994) (5.3451, -13.794) (5.3441, -13.7886) (5.3431, -13.7833) (5.3422, -13.778) (5.3412, -13.7728) (5.3402, -13.7676) (5.3392, -13.7624) (5.3382, -13.7573) (5.3372, -13.7523) (5.3363, -13.7473) (5.3353, -13.7423) (5.3343, -13.7374) (5.3333, -13.7325) (5.3323, -13.7277) (5.3313, -13.723) (5.3303, -13.7183) (5.3293, -13.7136) (5.3284, -13.709) (5.3274, -13.7044) (5.3264, -13.6999) (5.3254, -13.6954) (5.3244, -13.691) (5.3235, -13.6867) (5.3225, -13.6824) (5.3215, -13.6781) (5.3205, -13.6739) (5.3196, -13.6698) (5.3186, -13.6657) (5.3176, -13.6616) (5.3167, -13.6576) (5.3157, -13.6537) (5.3148, -13.6498) (5.3138, -13.646) (5.3129, -13.6422) (5.312, -13.6385) (5.3111, -13.6348) (5.3101, -13.6312) (5.3092, -13.6276) (5.3083, -13.6241) (5.3074, -13.6207) (5.3065, -13.6173) (5.3056, -13.614) (5.3047, -13.6107) (5.3039, -13.6075) (5.303, -13.6043) (5.3022, -13.6012) (5.3013, -13.5982) (5.3005, -13.5952) (5.2997, -13.5923) (5.2988, -13.5894) (5.298, -13.5866) (5.2972, -13.5839) (5.2965, -13.5812) (5.2957, -13.5786) (5.2949, -13.576) (5.2942, -13.5735) (5.2935, -13.5711) (5.2927, -13.5687) (5.292, -13.5664) (5.2913, -13.5641) (5.2907, -13.5619) (5.29, -13.5598) (5.2893, -13.5578) (5.2887, -13.5558) (5.2881, -13.5539) (5.2875, -13.552) (5.2869, -13.5502) (5.2863, -13.5485) (5.2858, -13.5468) (5.2853, -13.5452) (5.2848, -13.5437) (5.2843, -13.5423) (5.2838, -13.5409) (5.2833, -13.5396) (5.2829, -13.5383) (5.2825, -13.5372) (5.2821, -13.5361) (5.2818, -13.5351) (5.2814, -13.5341) (5.2811, -13.5332) (5.2808, -13.5324) (5.2805, -13.5317) (5.2803, -13.531) (5.2801, -13.5305) (5.2799, -13.53) (5.2798, -13.5296) (5.2797, -13.5294) (5.2796, -13.5293) (5.2796, -13.5292) knots -1 -1 -1 -1 -1 -1 -0.99583333 -0.99166667 -0.9875 -0.98333333 -0.97916667 -0.975 -0.97083333 -0.96666667 -0.9625 -0.95833333 -0.95416667 -0.95 -0.94583333 -0.94166667 -0.9375 -0.93333333 -0.92916667 -0.925 -0.92083333 -0.91666667 -0.9125 -0.90833333 -0.90416667 -0.9 -0.89583333 -0.89166667 -0.8875 -0.88333333 -0.87916667 -0.875 -0.87083333 -0.86666667 -0.8625 -0.85833333 -0.85416667 -0.85 -0.84583333 -0.84166667 -0.8375 -0.83333333 -0.82916667 -0.825 -0.82083333 -0.81666667 -0.8125 -0.80833333 -0.80416667 -0.8 -0.79583333 -0.79166667 -0.7875 -0.78333333 -0.77916667 -0.775 -0.77083333 -0.76666667 -0.7625 -0.75833333 -0.75416667 -0.75 -0.74583333 -0.74166667 -0.7375 -0.73333333 -0.72916667 -0.725 -0.72083333 -0.71666667 -0.7125 -0.70833333 -0.70416667 -0.7 -0.69583333 -0.69166667 -0.6875 -0.68333333 -0.67916667 -0.675 -0.67083333 -0.66666667 -0.6625 -0.65833333 -0.65416667 -0.65 -0.64583333 -0.64166667 -0.6375 -0.63333333 -0.62916667 -0.625 -0.62083333 -0.61666667 -0.6125 -0.60833333 -0.60416667 -0.6 -0.59583333 -0.59166667 -0.5875 -0.58333333 -0.57916667 -0.575 -0.57083333 -0.56666667 -0.5625 -0.55833333 -0.55416667 -0.55 -0.54583333 -0.54166667 -0.5375 -0.53333333 -0.52916667 -0.525 -0.52083333 -0.51666667 -0.5125 -0.50833333 -0.50416667 -0.5 -0.49583333 -0.49166667 -0.4875 -0.48333333 -0.47916667 -0.475 -0.47083333 -0.46666667 -0.4625 -0.45833333 -0.45416667 -0.45 -0.44583333 -0.44166667 -0.4375 -0.43333333 -0.42916667 -0.425 -0.42083333 -0.41666667 -0.4125 -0.40833333 -0.40416667 -0.4 -0.39583333 -0.39166667 -0.3875 -0.38333333 -0.37916667 -0.375 -0.37083333 -0.36666667 -0.3625 -0.35833333 -0.35416667 -0.35 -0.34583333 -0.34166667 -0.3375 -0.33333333 -0.32916667 -0.325 -0.32083333 -0.31666667 -0.3125 -0.30833333 -0.30416667 -0.3 -0.29583333 -0.29166667 -0.2875 -0.28333333 -0.27916667 -0.275 -0.27083333 -0.26666667 -0.2625 -0.25833333 -0.25416667 -0.25 -0.24583333 -0.24166667 -0.2375 -0.23333333 -0.22916667 -0.225 -0.22083333 -0.21666667 -0.2125 -0.20833333 -0.20416667 -0.2 -0.19583333 -0.19166667 -0.1875 -0.18333333 -0.17916667 -0.175 -0.17083333 -0.16666667 -0.1625 -0.15833333 -0.15416667 -0.15 -0.14583333 -0.14166667 -0.1375 -0.13333333 -0.12916667 -0.125 -0.12083333 -0.11666667 -0.1125 -0.10833333 -0.10416667 -0.1 -0.09583333 -0.09166667 -0.0875 -0.08333333 -0.07916667 -0.075 -0.07083333 -0.06666667 -0.0625 -0.05833333 -0.05416667 -0.05 -0.04583333 -0.04166667 -0.0375 -0.03333333 -0.02916667 -0.025 -0.02083333 -0.01666667 -0.0125 -0.00833333 -0.00416667 0 0 0 0 0 0
  arc A31 (2.2262, -13.5686) -> (3.4851, -13.301) centre (0, 0) ccw
  arc A32 (-0.6435, -13.7349) -> (0.6435, -13.7349) centre (0, 0) ccw
  line L68 (-13.5924, -2.0756) -> (-14.3558, -2.1922)
  arc A33 (1.2166, -15.9537) -> (2.127, -15.858) centre (0, 0) ccw
  circle A34 centre (0, -10) radius 1.7
  spline S23 degree 5 poles (12.2236, 7.8421) (12.2236, 7.8421) (12.2237, 7.8422) (12.2239, 7.8423) (12.2242, 7.8425) (12.2247, 7.8428) (12.2252, 7.8431) (12.2258, 7.8435) (12.2264, 7.844) (12.2271, 7.8445) (12.2279, 7.845) (12.2287, 7.8455) (12.2296, 7.8462) (12.2306, 7.8468) (12.2316, 7.8475) (12.2327, 7.8483) (12.2338, 7.8491) (12.235, 7.8499) (12.2363, 7.8508) (12.2376, 7.8517) (12.2389, 7.8527) (12.2403, 7.8537) (12.2418, 7.8548) (12.2433, 7.8559) (12.2449, 7.857) (12.2465, 7.8582) (12.2482, 7.8595) (12.25, 7.8608) (12.2517, 7.8621) (12.2536, 7.8634) (12.2555, 7.8649) (12.2574, 7.8663) (12.2594, 7.8678) (12.2614, 7.8693) (12.2635, 7.8709) (12.2656, 7.8726) (12.2677, 7.8742) (12.27, 7.8759) (12.2722, 7.8777) (12.2745, 7.8795) (12.2769, 7.8813) (12.2792, 7.8832) (12.2817, 7.8851) (12.2841, 7.8871) (12.2867, 7.8891) (12.2892, 7.8911) (12.2918, 7.8932) (12.2944, 7.8954) (12.2971, 7.8975) (12.2998, 7.8998) (12.3026, 7.902) (12.3054, 7.9043) (12.3082, 7.9066) (12.3111, 7.909) (12.314, 7.9115) (12.3169, 7.9139) (12.3199, 7.9164) (12.3229, 7.919) (12.326, 7.9216) (12.329, 7.9242) (12.3322, 7.9268) (12.3353, 7.9296) (12.3385, 7.9323) (12.3417, 7.9351) (12.345, 7.9379) (12.3483, 7.9408) (12.3516, 7.9437) (12.3549, 7.9467) (12.3583, 7.9496) (12.3617, 7.9527) (12.3652, 7.9558) (12.3687, 7.9589) (12.3722, 7.962) (12.3757, 7.9652) (12.3793, 7.9684) (12.3829, 7.9717) (12.3865, 7.975) (12.3902, 7.9784) (12.3938, 7.9818) (12.3976, 7.9852) (12.4013, 7.9887) (12.4051, 7.9922) (12.4089, 7.9957) (12.4127, 7.9993) (12.4165, 8.0029) (12.4204, 8.0066) (12.4243, 8.0103) (12.4282, 8.014) (12.4322, 8.0178) (12.4361, 8.0216) (12.4401, 8.0255) (12.4442, 8.0294) (12.4482, 8.0333) (12.4523, 8.0373) (12.4564, 8.0413) (12.4605, 8.0454) (12.4647, 8.0495) (12.4688, 8.0536) (12.473, 8.0578) (12.4772, 8.062) (12.4815, 8.0662) (12.4857, 8.0705) (12.49, 8.0748) (12.4943, 8.0792) (12.4986, 8.0836) (12.5029, 8.088) (12.5073, 8.0925) (12.5117, 8.097) (12.5161, 8.1015) (12.5205, 8.1061) (12.5249, 8.1107) (12.5294, 8.1154) (12.5339, 8.1201) (12.5384, 8.1248) (12.5429, 8.1296) (12.5474, 8.1344) (12.552, 8.1393) (12.5565, 8.1441) (12.5611, 8.1491) (12.5657, 8.154) (12.5703, 8.159) (12.575, 8.1641) (12.5796, 8.1691) (12.5843, 8.1742) (12.589, 8.1794) (12.5937, 8.1846) (12.5984, 8.1898) (12.6032, 8.195) (12.6079, 8.2003) (12.6127, 8.2056) (12.6175, 8.211) (12.6223, 8.2164) (12.6271, 8.2218) (12.6319, 8.2273) (12.6367, 8.2328) (12.6416, 8.2384) (12.6465, 8.2439) (12.6513, 8.2496) (12.6562, 8.2552) (12.6612, 8.2609) (12.6661, 8.2666) (12.671, 8.2724) (12.676, 8.2782) (12.6809, 8.284) (12.6859, 8.2899) (12.6909, 8.2958) (12.6959, 8.3017) (12.7009, 8.3077) (12.7059, 8.3137) (12.7109, 8.3198) (12.716, 8.3259) (12.721, 8.332) (12.7261, 8.3381) (12.7312, 8.3443) (12.7363, 8.3505) (12.7414, 8.3568) (12.7465, 8.3631) (12.7516, 8.3694) (12.7567, 8.3758) (12.7619, 8.3822) (12.767, 8.3886) (12.7722, 8.3951) (12.7773, 8.4016) (12.7825, 8.4081) (12.7877, 8.4147) (12.7929, 8.4213) (12.7981, 8.4279) (12.8033, 8.4346) (12.8085, 8.4413) (12.8138, 8.4481) (12.819, 8.4549) (12.8242, 8.4617) (12.8295, 8.4685) (12.8347, 8.4754) (12.84, 8.4823) (12.8453, 8.4893) (12.8506, 8.4963) (12.8558, 8.5033) (12.8611, 8.5103) (12.8664, 8.5174) (12.8718, 8.5246) (12.8771, 8.5317) (12.8824, 8.5389) (12.8877, 8.5461) (12.893, 8.5534) (12.8984, 8.5607) (12.9037, 8.568) (12.9091, 8.5754) (12.9144, 8.5827) (12.9198, 8.5902) (12.9252, 8.5976) (12.9305, 8.6051) (12.9359, 8.6126) (12.9413, 8.6202) (12.9467, 8.6278) (12.9521, 8.6354) (12.9574, 8.6431) (12.9628, 8.6508) (12.9682, 8.6585) (12.9736, 8.6663) (12.9791, 8.6741) (12.9845, 8.6819) (12.9899, 8.6897) (12.9953, 8.6976) (13.0007, 8.7055) (13.0062, 8.7135) (13.0116, 8.7215) (13.017, 8.7295) (13.0224, 8.7376) (13.0279, 8.7456) (13.0333, 8.7538) (13.0388, 8.7619) (13.0442, 8.7701) (13.0497, 8.7783) (13.0551, 8.7866) (13.0606, 8.7948) (13.066, 8.8032) (13.0715, 8.8115) (13.0769, 8.8199) (13.0824, 8.8283) (13.0878, 8.8367) (13.0933, 8.8452) (13.0988, 8.8537) (13.1042, 8.8622) (13.1097, 8.8708) (13.1151, 8.8794) (13.1206, 8.888) (13.1261, 8.8967) (13.1315, 8.9054) (13.137, 8.9141) (13.1425, 8.9229) (13.1479, 8.9317) (13.1534, 8.9405) (13.1589, 8.9493) (13.1643, 8.9582) (13.1698, 8.9671) (13.1752, 8.9761) (13.1807, 8.9851) (13.1862, 8.9941) (13.1916, 9.0031) (13.1971, 9.0122) (13.2015, 9.0195) (13.2047, 9.0249) (13.2069, 9.0286) (13.208, 9.0304) knots 0 0 0 0 0 0 0.00416667 0.00833333 0.0125 0.01666667 0.02083333 0.025 0.02916667 0.03333333 0.0375 0.04166667 0.04583333 0.05 0.05416667 0.05833333 0.0625 0.06666667 0.07083333 0.075 0.07916667 0.08333333 0.0875 0.09166667 0.09583333 0.1 0.10416667 0.10833333 0.1125 0.11666667 0.12083333 0.125 0.12916667 0.13333333 0.1375 0.14166667 0.14583333 0.15 0.15416667 0.15833333 0.1625 0.16666667 0.17083333 0.175 0.17916667 0.18333333 0.1875 0.19166667 0.19583333 0.2 0.20416667 0.20833333 0.2125 0.21666667 0.22083333 0.225 0.22916667 0.23333333 0.2375 0.24166667 0.24583333 0.25 0.25416667 0.25833333 0.2625 0.26666667 0.27083333 0.275 0.27916667 0.28333333 0.2875 0.29166667 0.29583333 0.3 0.30416667 0.30833333 0.3125 0.31666667 0.32083333 0.325 0.32916667 0.33333333 0.3375 0.34166667 0.34583333 0.35 0.35416667 0.35833333 0.3625 0.36666667 0.37083333 0.375 0.37916667 0.38333333 0.3875 0.39166667 0.39583333 0.4 0.40416667 0.40833333 0.4125 0.41666667 0.42083333 0.425 0.42916667 0.43333333 0.4375 0.44166667 0.44583333 0.45 0.45416667 0.45833333 0.4625 0.46666667 0.47083333 0.475 0.47916667 0.48333333 0.4875 0.49166667 0.49583333 0.5 0.50416667 0.50833333 0.5125 0.51666667 0.52083333 0.525 0.52916667 0.53333333 0.5375 0.54166667 0.54583333 0.55 0.55416667 0.55833333 0.5625 0.56666667 0.57083333 0.575 0.57916667 0.58333333 0.5875 0.59166667 0.59583333 0.6 0.60416667 0.60833333 0.6125 0.61666667 0.62083333 0.625 0.62916667 0.63333333 0.6375 0.64166667 0.64583333 0.65 0.65416667 0.65833333 0.6625 0.66666667 0.67083333 0.675 0.67916667 0.68333333 0.6875 0.69166667 0.69583333 0.7 0.70416667 0.70833333 0.7125 0.71666667 0.72083333 0.725 0.72916667 0.73333333 0.7375 0.74166667 0.74583333 0.75 0.75416667 0.75833333 0.7625 0.76666667 0.77083333 0.775 0.77916667 0.78333333 0.7875 0.79166667 0.79583333 0.8 0.80416667 0.80833333 0.8125 0.81666667 0.82083333 0.825 0.82916667 0.83333333 0.8375 0.84166667 0.84583333 0.85 0.85416667 0.85833333 0.8625 0.86666667 0.87083333 0.875 0.87916667 0.88333333 0.8875 0.89166667 0.89583333 0.9 0.90416667 0.90833333 0.9125 0.91666667 0.92083333 0.925 0.92916667 0.93333333 0.9375 0.94166667 0.94583333 0.95 0.95416667 0.95833333 0.9625 0.96666667 0.97083333 0.975 0.97916667 0.98333333 0.9875 0.99166667 0.99583333 1 1 1 1 1 1
  line L69 (-14.007, -3.8365) -> (-14.0063, -3.8363)
  arc A35 (7.6003, -14.0796) -> (8.3931, -13.6219) centre (0, 0) ccw
  line L70 (-14.4985, -0.8405) -> (-14.4979, -0.8404)
  line L71 (5.2794, -13.5286) -> (4.9987, -12.8092)
  line L72 (-14.3558, -2.1922) -> (-14.3564, -2.1923)
  spline S24 degree 5 poles (7.6003, 14.0796) (7.5986, 14.0783) (7.5952, 14.0758) (7.5901, 14.0719) (7.5833, 14.0668) (7.5749, 14.0604) (7.5665, 14.0541) (7.5581, 14.0477) (7.5497, 14.0413) (7.5414, 14.035) (7.5331, 14.0286) (7.5248, 14.0222) (7.5166, 14.0159) (7.5084, 14.0095) (7.5002, 14.0032) (7.4921, 13.9968) (7.484, 13.9905) (7.4759, 13.9841) (7.4679, 13.9778) (7.4599, 13.9714) (7.4519, 13.9651) (7.4439, 13.9588) (7.436, 13.9525) (7.4281, 13.9461) (7.4203, 13.9398) (7.4124, 13.9335) (7.4046, 13.9272) (7.3969, 13.9209) (7.3892, 13.9146) (7.3815, 13.9083) (7.3738, 13.902) (7.3662, 13.8958) (7.3586, 13.8895) (7.351, 13.8832) (7.3435, 13.8769) (7.336, 13.8707) (7.3285, 13.8644) (7.321, 13.8582) (7.3136, 13.8519) (7.3063, 13.8457) (7.2989, 13.8395) (7.2916, 13.8333) (7.2843, 13.827) (7.2771, 13.8208) (7.2699, 13.8146) (7.2627, 13.8084) (7.2555, 13.8023) (7.2484, 13.7961) (7.2413, 13.7899) (7.2343, 13.7837) (7.2272, 13.7776) (7.2203, 13.7714) (7.2133, 13.7653) (7.2064, 13.7592) (7.1995, 13.753) (7.1926, 13.7469) (7.1858, 13.7408) (7.179, 13.7347) (7.1723, 13.7286) (7.1655, 13.7226) (7.1588, 13.7165) (7.1522, 13.7104) (7.1455, 13.7044) (7.1389, 13.6983) (7.1324, 13.6923) (7.1259, 13.6863) (7.1194, 13.6803) (7.1129, 13.6743) (7.1065, 13.6683) (7.1001, 13.6623) (7.0937, 13.6563) (7.0874, 13.6504) (7.0811, 13.6444) (7.0748, 13.6385) (7.0686, 13.6325) (7.0624, 13.6266) (7.0562, 13.6207) (7.0501, 13.6148) (7.044, 13.6089) (7.0379, 13.6031) (7.0319, 13.5972) (7.0259, 13.5914) (7.02, 13.5855) (7.014, 13.5797) (7.0081, 13.5739) (7.0023, 13.5681) (6.9965, 13.5624) (6.9907, 13.5566) (6.9849, 13.5508) (6.9792, 13.5451) (6.9735, 13.5394) (6.9678, 13.5337) (6.9622, 13.528) (6.9566, 13.5223) (6.9511, 13.5166) (6.9455, 13.511) (6.94, 13.5053) (6.9346, 13.4997) (6.9292, 13.4941) (6.9238, 13.4885) (6.9184, 13.4829) (6.9131, 13.4774) (6.9078, 13.4718) (6.9026, 13.4663) (6.8974, 13.4608) (6.8922, 13.4553) (6.8871, 13.4498) (6.8819, 13.4444) (6.8769, 13.4389) (6.8718, 13.4335) (6.8668, 13.4281) (6.8618, 13.4227) (6.8569, 13.4173) (6.852, 13.412) (6.8471, 13.4066) (6.8423, 13.4013) (6.8375, 13.396) (6.8327, 13.3907) (6.828, 13.3855) (6.8233, 13.3802) (6.8187, 13.375) (6.814, 13.3698) (6.8094, 13.3646) (6.8049, 13.3595) (6.8004, 13.3543) (6.7959, 13.3492) (6.7914, 13.3441) (6.787, 13.339) (6.7826, 13.334) (6.7783, 13.329) (6.774, 13.3239) (6.7697, 13.319) (6.7655, 13.314) (6.7613, 13.309) (6.7571, 13.3041) (6.753, 13.2992) (6.7489, 13.2944) (6.7448, 13.2895) (6.7408, 13.2847) (6.7368, 13.2799) (6.7328, 13.2751) (6.7289, 13.2703) (6.725, 13.2656) (6.7212, 13.2609) (6.7174, 13.2562) (6.7136, 13.2516) (6.7098, 13.2469) (6.7061, 13.2423) (6.7025, 13.2378) (6.6988, 13.2332) (6.6952, 13.2287) (6.6917, 13.2242) (6.6881, 13.2197) (6.6846, 13.2153) (6.6812, 13.2109) (6.6778, 13.2065) (6.6744, 13.2022) (6.671, 13.1978) (6.6677, 13.1935) (6.6644, 13.1893) (6.6612, 13.185) (6.658, 13.1808) (6.6548, 13.1767) (6.6517, 13.1725) (6.6486, 13.1684) (6.6455, 13.1643) (6.6425, 13.1603) (6.6395, 13.1563) (6.6366, 13.1523) (6.6337, 13.1483) (6.6308, 13.1444) (6.628, 13.1405) (6.6252, 13.1367) (6.6224, 13.1328) (6.6197, 13.1291) (6.617, 13.1253) (6.6143, 13.1216) (6.6117, 13.1179) (6.6091, 13.1143) (6.6065, 13.1107) (6.604, 13.1071) (6.6016, 13.1036) (6.5991, 13.1001) (6.5967, 13.0966) (6.5944, 13.0932) (6.592, 13.0898) (6.5897, 13.0865) (6.5875, 13.0832) (6.5853, 13.0799) (6.5831, 13.0767) (6.581, 13.0735) (6.5788, 13.0703) (6.5768, 13.0672) (6.5747, 13.0642) (6.5728, 13.0612) (6.5708, 13.0582) (6.5689, 13.0553) (6.567, 13.0524) (6.5651, 13.0495) (6.5633, 13.0467) (6.5616, 13.044) (6.5598, 13.0413) (6.5581, 13.0386) (6.5565, 13.036) (6.5549, 13.0334) (6.5533, 13.0309) (6.5517, 13.0284) (6.5502, 13.026) (6.5488, 13.0236) (6.5473, 13.0213) (6.5459, 13.019) (6.5446, 13.0168) (6.5433, 13.0146) (6.542, 13.0125) (6.5407, 13.0104) (6.5395, 13.0084) (6.5384, 13.0064) (6.5372, 13.0045) (6.5361, 13.0027) (6.5351, 13.0009) (6.5341, 12.9991) (6.5331, 12.9974) (6.5321, 12.9958) (6.5312, 12.9942) (6.5304, 12.9927) (6.5295, 12.9913) (6.5288, 12.9899) (6.528, 12.9885) (6.5273, 12.9873) (6.5266, 12.986) (6.526, 12.9849) (6.5254, 12.9838) (6.5248, 12.9828) (6.5243, 12.9818) (6.5238, 12.9809) (6.5234, 12.9801) (6.523, 12.9794) (6.5226, 12.9787) (6.5223, 12.9781) (6.522, 12.9775) (6.5218, 12.977) (6.5216, 12.9767) (6.5215, 12.9765) (6.5214, 12.9764) (6.5214, 12.9763) knots -1 -1 -1 -1 -1 -1 -0.99583333 -0.99166667 -0.9875 -0.98333333 -0.97916667 -0.975 -0.97083333 -0.96666667 -0.9625 -0.95833333 -0.95416667 -0.95 -0.94583333 -0.94166667 -0.9375 -0.93333333 -0.92916667 -0.925 -0.92083333 -0.91666667 -0.9125 -0.90833333 -0.90416667 -0.9 -0.89583333 -0.89166667 -0.8875 -0.88333333 -0.87916667 -0.875 -0.87083333 -0.86666667 -0.8625 -0.85833333 -0.85416667 -0.85 -0.84583333 -0.84166667 -0.8375 -0.83333333 -0.82916667 -0.825 -0.82083333 -0.81666667 -0.8125 -0.80833333 -0.80416667 -0.8 -0.79583333 -0.79166667 -0.7875 -0.78333333 -0.77916667 -0.775 -0.77083333 -0.76666667 -0.7625 -0.75833333 -0.75416667 -0.75 -0.74583333 -0.74166667 -0.7375 -0.73333333 -0.72916667 -0.725 -0.72083333 -0.71666667 -0.7125 -0.70833333 -0.70416667 -0.7 -0.69583333 -0.69166667 -0.6875 -0.68333333 -0.67916667 -0.675 -0.67083333 -0.66666667 -0.6625 -0.65833333 -0.65416667 -0.65 -0.64583333 -0.64166667 -0.6375 -0.63333333 -0.62916667 -0.625 -0.62083333 -0.61666667 -0.6125 -0.60833333 -0.60416667 -0.6 -0.59583333 -0.59166667 -0.5875 -0.58333333 -0.57916667 -0.575 -0.57083333 -0.56666667 -0.5625 -0.55833333 -0.55416667 -0.55 -0.54583333 -0.54166667 -0.5375 -0.53333333 -0.52916667 -0.525 -0.52083333 -0.51666667 -0.5125 -0.50833333 -0.50416667 -0.5 -0.49583333 -0.49166667 -0.4875 -0.48333333 -0.47916667 -0.475 -0.47083333 -0.46666667 -0.4625 -0.45833333 -0.45416667 -0.45 -0.44583333 -0.44166667 -0.4375 -0.43333333 -0.42916667 -0.425 -0.42083333 -0.41666667 -0.4125 -0.40833333 -0.40416667 -0.4 -0.39583333 -0.39166667 -0.3875 -0.38333333 -0.37916667 -0.375 -0.37083333 -0.36666667 -0.3625 -0.35833333 -0.35416667 -0.35 -0.34583333 -0.34166667 -0.3375 -0.33333333 -0.32916667 -0.325 -0.32083333 -0.31666667 -0.3125 -0.30833333 -0.30416667 -0.3 -0.29583333 -0.29166667 -0.2875 -0.28333333 -0.27916667 -0.275 -0.27083333 -0.26666667 -0.2625 -0.25833333 -0.25416667 -0.25 -0.24583333 -0.24166667 -0.2375 -0.23333333 -0.22916667 -0.225 -0.22083333 -0.21666667 -0.2125 -0.20833333 -0.20416667 -0.2 -0.19583333 -0.19166667 -0.1875 -0.18333333 -0.17916667 -0.175 -0.17083333 -0.16666667 -0.1625 -0.15833333 -0.15416667 -0.15 -0.14583333 -0.14166667 -0.1375 -0.13333333 -0.12916667 -0.125 -0.12083333 -0.11666667 -0.1125 -0.10833333 -0.10416667 -0.1 -0.09583333 -0.09166667 -0.0875 -0.08333333 -0.07916667 -0.075 -0.07083333 -0.06666667 -0.0625 -0.05833333 -0.05416667 -0.05 -0.04583333 -0.04166667 -0.0375 -0.03333333 -0.02916667 -0.025 -0.02083333 -0.01666667 -0.0125 -0.00833333 -0.00416667 0 0 0 0 0 0
  line L73 (9.0764, -11.3364) -> (9.0768, -11.3369)
  arc A36 (7.5526, -11.49) -> (8.5938, -10.7336) centre (0, 0) ccw
  line L74 (6.1743, -12.2858) -> (6.5211, -12.9757)
  line L75 (8.5938, -10.7336) -> (9.0764, -11.3364)
  line L76 (7.9771, -12.1359) -> (7.9768, -12.1353)